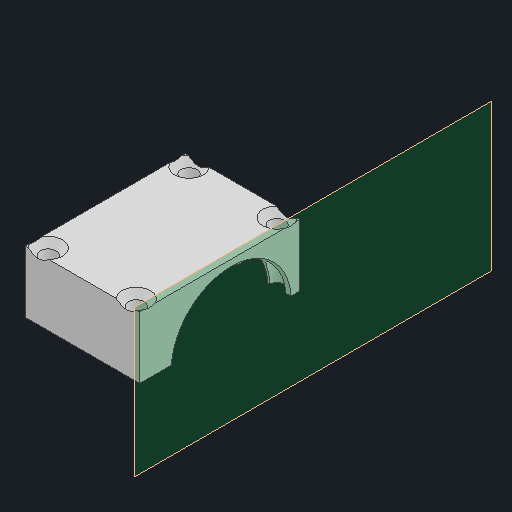
# Autodesk Inventor part: right_motor_ceil
Saved by Autodesk Inventor 2023 (Build 270158000, 158)
## iProperties
Created: 2024-04-14
Part Number: right_motor_ceil
Material: Generic
Document SubType Name: Modeling
Designer: szymo
Density: 1 g/cm^3
Appearance: Default
Mass: 5.68525 g
Surface Area: 39.9692 cm^2
Volume: 5.68525 cm^3
Author: szymo
Autodesk Inventor part; units mm, degrees
ref_plane "YZ Plane" through (0, 0, 0) normal (1, 0, 0) x (0, 1, 0)
ref_plane "XZ Plane" through (0, 0, 0) normal (0, 1, 0) x (-1, 0, 0)
ref_plane "XY Plane" through (0, 0, 0) normal (0, 0, 1) x (1, 0, 0)
ref_plane "Work Plane1" through (44.4579, -56.5766, -83.6387) normal (-1, 0, 0) x (0, 0, 1)
sketch "Sketch1" plane through (44.4579, -56.5766, -83.6387) normal (-1, 0, 0) x (0, 0, 1)
  line L0 (92.9615, 0) -> (92.9615, 14.375) projected
  line L1 (92.9615, 14.375) -> (97.4615, 14.375) projected
  arc A0 (97.4615, 14.375) -> (124.7885, 14.375) centre (111.125, 15.375) ccw projected
  line L2 (124.7885, 14.375) -> (129.5, 14.375) projected
  line L3 (129.5, 14.375) -> (129.5, 30.5) projected
  line L4 (52.8275, 30.5) -> (129.5, 30.5) projected
  line L5 (52.8275, 10) -> (59.8275, 10) projected
  line L6 (59.8275, 10) -> (59.8275, 0) projected
  line L7 (59.8275, 0) -> (92.9615, 0) projected
  line L8 (119.625, 13.875) -> (120.125, 13.875) projected
  line L9 (120.125, 13.875) -> (120.125, 16.875) projected
  line L10 (120.125, 16.875) -> (119.625, 16.875) projected
  line L11 (119.625, 16.875) -> (119.625, 13.875) projected
  line L12 (97.125, 16.875) -> (96.625, 16.875) projected
  line L13 (96.625, 16.875) -> (96.625, 13.875) projected
  line L14 (96.625, 13.875) -> (97.125, 13.875) projected
  line L15 (97.125, 13.875) -> (97.125, 16.875) projected
  circle A1 centre (108.625, 15.375) radius 5 projected
  circle A2 centre (108.625, 15.375) radius 13.7 projected
  line L16 (92.9615, 14.375) -> (129.5, 14.375)
  line L17 (129.5, 14.375) -> (129.5, 30.5)
  line L18 (129.5, 30.5) -> (92.9615, 30.5)
  line L19 (92.9615, 30.5) -> (92.9615, 14.375)
  line L20 (92.9615, 16.375) -> (129.5, 16.375)
  line L21 (52.8275, 30.5) -> (23, 13.2791) projected
  line L22 (23, 13.2791) -> (23, 9.2376) projected
  line L23 (23, 9.2376) -> (23, 0) projected
  line L24 (23, 0) -> (52.8275, 0) projected
  line L25 (52.8275, 0) -> (52.8275, 10) projected
  point P0 (83.6387, 56.5766)
  point P1 (94.9615, 16.375)
  point P2 (122.2885, 16.375)
  point P3 (92.9615, 30.5)
  dimension "d0" = 2
  constraints: 10 end point, 2 horizontal, 2 parallel, 2 point on line, 1 perpendicular, 1 other
  measures "d0" distance from line of L20 L0.end
ref_plane "Work Plane2" through (18.3579, -55.5766, 10.6113) normal (1, 0, 0) x (0, 1, 0)
extrude "Extrusion1" add sketch "Sketch1" along normal up to surface (26.1 mm away) contours L19 L4 L3 L20 A2
sketch "Sketch2" plane through (44.4579, -26.0766, 45.8613) normal (0, 1, 0) x (1, 0, 0)
  line L0 (-26.1, 0) -> (-26.1, 4.7115) projected
  line L1 (0, 0) -> (-26.1, 0) projected
  line L2 (0, 4.7115) -> (0, 0) projected
  line L3 (0, 4.7115) -> (-26.1, 4.7115) projected
  line L4 (-26.1, 32.0385) -> (-26.1, 36.5385) projected
  line L5 (0, 32.0385) -> (-26.1, 32.0385) projected
  line L6 (0, 36.5385) -> (0, 32.0385) projected
  line L7 (0, 36.5385) -> (-26.1, 36.5385) projected
  line L8 (-3, 34.3385) -> (-23.1, 34.3385)
  line L9 (-23.1, 34.3385) -> (-23.1, 2.2)
  line L10 (-23.1, 2.2) -> (-3, 2.2)
  line L11 (-3, 2.2) -> (-3, 34.3385)
  point P0 (-44.4579, 45.8613)
  dimension "d3" = 2.2
  dimension "d4" = 2.2
  dimension "d5" = 3
  dimension "d6" = 3
  constraints: 8 end point, 4 coincident, 2 parallel, 1 horizontal, 1 perpendicular
  measures "d3" distance between parallel lines of L7 L8
  measures "d4" distance between parallel lines of L10 L1
  measures "d5" distance between parallel lines of L2 L11
  measures "d6" distance between parallel lines of L4 L9
hole "Hole1" at (41.4579, -26.0766, 11.5229) at (41.4579, -26.0766, 43.6613) at (21.3579, -26.0766, 43.6613) at (21.3579, -26.0766, 11.5229) direction (0, -1, 0) diameter 3.6 end through all countersink diameter 6.5 countersink angle 90
sketch "Sketch3" plane through (44.4579, -40.2016, 9.3229) normal (0, 0, -1) x (-1, 0, 0)
  line L0 (0, 14.125) -> (0.6078, 14.125)
  line L1 (0, 14.125) -> (0, 0)
  line L2 (0, 0) -> (26.1, 0)
  line L3 (26.1, 14.125) -> (26.1, 0)
  line L4 (25.4922, 14.125) -> (26.1, 14.125)
  line L5 (5.3922, 14.125) -> (20.7078, 14.125)
  line L6 (12.3, 0.5) -> (12.3, -2.5)
  line L7 (12.3, 0.5) -> (6.3, 0.5)
  line L8 (6.3, -2.5) -> (6.3, 0.5)
  line L9 (12.3, -2.5) -> (6.3, -2.5)
  line L10 (12.3, -14.7) -> (12.3, 12.7)
  line L11 (5.1794, -2) -> (20.9206, -2)
  line L12 (4.7748, -16.375) -> (21.3252, -16.375)
  line L13 (12.3, -2) -> (5.3, -2)
  line L14 (5.3, -2) -> (5.3, 5)
  line L15 (5.3, 5) -> (12.3, 5)
  line L16 (12.3, 5) -> (12.3, -2)
  spline S0 degree 2 poles (20.9206, -2) (21.1431, -2.2205) (21.3252, -2.4) knots 0 0 0 1 1 1 weights 1 1.096715 1.190476
  spline S1 degree 2 poles (4.7748, -2.4) (4.9569, -2.2205) (5.1794, -2) knots 0 0 0 1 1 1 weights 1.190476 1.096715 1
  line L17 (4.7748, -2.4) -> (4.7748, -16.375)
  line L18 (21.3252, -16.375) -> (21.3252, -2.4)
  point P0 (44.4579, 40.2016)
  point P1 (12.3, 5)
  point P2 (5.3, -2)
  dimension "d14" = 7
  dimension "d15" = 7
  constraints: 8 end point, 2 horizontal alignment, 2 parallel, 2 point on line, 1 horizontal, 1 perpendicular
  measures "d14" distance of L14.end L15.end
  measures "d15" distance of L13.end L14.end
extrude "Extrusion2" cut sketch "Sketch3" against normal blind 10 contours L14 L15 L10 L7 L8 L2 | L2 L8 L11 L14 | L8 L7 L6 L2 | L2 L6 L11 L8
body "Solid1"
